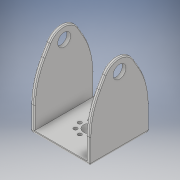
# Autodesk Inventor part: Wheel Case
Saved by Autodesk Inventor 2019 (Build 230136000, 136)
## iProperties
Created: 2018-12-01
Part Number: Wheel Case
Material: Generic
Document SubType Name: Modeling
Designer: Ashley
Density: 1 g/cm^3
Appearance: Default
Author: Ashley
Autodesk Inventor part; units mm, degrees
ref_plane "YZ Plane" through (0, 0, 0) normal (1, 0, 0) x (0, 1, 0)
ref_plane "XZ Plane" through (0, 0, 0) normal (0, 1, 0) x (-1, 0, 0)
ref_plane "XY Plane" through (0, 0, 0) normal (0, 0, 1) x (1, 0, 0)
sketch "Sketch1" plane through (0, 0, 0) normal (0, 1, 0) x (-1, 0, 0)
  line L0 (32.5, 32.5) -> (-32.5, 32.5)
  line L1 (-32.5, 32.5) -> (-32.5, -32.5)
  line L2 (-32.5, -32.5) -> (32.5, -32.5)
  line L3 (32.5, -32.5) -> (32.5, 32.5)
  line L4 (32.5, 32.5) -> (-32.5, -32.5) construction
  line L5 (-32.5, 32.5) -> (32.5, -32.5) construction
  point P0 (0, 0)
  dimension "d0" = 65
  dimension "d1" = 65
  constraints: 12 end point, 2 midpoint, 2 parallel, 1 horizontal, 1 perpendicular
  measures "d0" distance of L1.end L2.end
  measures "d1" distance of L0.end L1.end
extrude "Top Base Extrusion" add sketch "Sketch1" along normal blind 4
sketch "Sketch2" plane through (0, 4, 0) normal (0, 1, 0) x (1, 0, 0)
  line L0 (-32.5, -32.5) -> (32.5, -32.5) construction
  line L1 (32.5, -32.5) -> (32.5, 32.5) construction
  line L2 (-32.5, 32.5) -> (-32.5, -32.5) construction
  line L3 (-32.5, 32.5) -> (-28.5, 32.5)
  line L4 (-28.5, 32.5) -> (-28.5, -32.5)
  line L5 (-28.5, -32.5) -> (-32.5, -32.5)
  line L6 (-32.5, -32.5) -> (-32.5, 32.5)
  line L7 (32.5, 32.5) -> (28.5, 32.5)
  line L8 (28.5, 32.5) -> (28.5, -32.5)
  line L9 (28.5, -32.5) -> (32.5, -32.5)
  line L10 (32.5, -32.5) -> (32.5, 32.5)
  point P0 (0, 0)
  dimension "d4" = 4
  dimension "d5" = 4
  constraints: 16 end point, 4 parallel, 2 horizontal, 2 perpendicular, 2 point on line
  measures "d4" distance between parallel lines of L4 L2
  measures "d5" distance between parallel lines of L1 L8
extrude "Side Extrusions" add sketch "Sketch2" along normal blind 83.6
sketch "Sketch3" plane through (32.5, 0, 32.5) normal (1, 0, 0) x (0, 0, -1)
  circle A0 centre (32.5, 74.5) radius 7.1
  point P0 (32.5, 0)
  dimension "d8" = 14.2
  dimension "d11" = 74.5
  constraints: 1 centre point
  measures "d8" diameter of A0
  measures "d11" distance of point (32.5, 0) A0.centre
extrude "Wheel Axel Hole" cut sketch "Sketch3" against normal up to surface (65 mm away)
sketch "Sketch4" plane through (0, 0, 0) normal (0, -1, 0) x (1, 0, 0)
  circle A0 centre (0, 0) radius 7.1
  circle A1 centre (0, 0) radius 16
  dimension "d16" = 14.2
  dimension "d17" = 32
  constraints: 2 centre point, 2 coincident
  measures "d16" diameter of A0
  measures "d17" diameter of A1
extrude "Chain Interferance Extrusion" add sketch "Sketch4" along normal blind 6
sketch "Sketch5" plane through (0, 0, 0) normal (0, -1, 0) x (1, 0, 0)
  circle A0 centre (0, 0) radius 7.1 construction
  circle A1 centre (0, 0) radius 7.1
  constraints: 1 centre point, 1 coincident, 1 concentric
extrude "Top Center Bearing Hole" cut sketch "Sketch5" against normal up to surface (4 mm away)
sketch "Sketch7" plane through (0, -6, 0) normal (0, -1, 0) x (1, 0, 0)
  circle A0 centre (0, 0) radius 7.1 construction
  circle A1 centre (0, 11.314) radius 2.05
  circle A2 centre (-8.0002, 8.0002) radius 2.05
  circle A3 centre (-11.314, 0) radius 2.05
  circle A4 centre (-8.0002, -8.0002) radius 2.05
  circle A5 centre (0, -11.314) radius 2.05
  circle A6 centre (8.0002, -8.0002) radius 2.05
  circle A7 centre (11.314, 0) radius 2.05
  circle A8 centre (8.0002, 8.0002) radius 2.05
  dimension "d23" = 4.1
  dimension "d24" = 11.314
  dimension "d27" = 360
  constraints: 8 centre point, 17 other
  measures "d23" diameter of A1
  measures "d24" distance of A0.centre A1.centre
extrude "Sprocket Screws Holes" cut sketch "Sketch7" against normal up to next
sketch "Sketch8" plane through (32.5, 0, 32.5) normal (1, 0, 0) x (0, 0, -1)
  line L0 (65, 0) -> (65, 87.6) construction
  line L1 (0, 87.6) -> (65, 87.6) construction
  line L2 (0, 0) -> (0, 87.6) construction
  line L3 (65, 49.2769) -> (42.8742, 87.6)
  line L4 (65, 87.6) -> (0, 87.6) construction
  line L5 (65, 49.2769) -> (109.2517, 49.2769) construction
  line L6 (0, 49.2769) -> (45.0213, 49.2769) construction
  line L7 (0, 49.2769) -> (44.4453, 49.2769) construction
  line L8 (0, 49.2769) -> (22.1258, 87.6)
  line L9 (65, 49.2769) -> (65, 87.6)
  line L10 (42.8742, 87.6) -> (65, 87.6)
  line L11 (22.1258, 87.6) -> (0, 87.6)
  line L12 (0, 49.2769) -> (0, 87.6)
  point P0 (32.5, 0)
  dimension "d32" = 120
  constraints: 18 end point, 4 point on line, 3 collinear, 3 horizontal, 1 equal length, 1 perpendicular
  measures "d32" angle of L5 L3
extrude "Extrusion7" cut sketch "Sketch8" against normal up to surface (65 mm away)
fillet "Fillet1" radius 80 4 edges at (30.5, 49.2769, 32.5) (-30.5, 49.2769, 32.5) (30.5, 49.2769, -32.5) (-30.5, 49.2769, -32.5)
fillet "Fillet2" radius 18 4 edges at (30.5, 87.6, 10.3742) (30.5, 87.6, -10.3742) (-30.5, 87.6, -10.3742) (-30.5, 87.6, 10.3742)
fillet "Fillet3" radius 3 4 edges at (0, 0, -32.5) (-32.5, 0, 0) (32.5, 0, 0) (0, 0, 32.5)
fillet "Fillet4" radius 3 1 edges at (-16, 0, 0)
fillet "Fillet5" radius 1 1 edges at (-16, -6, 0)
fillet "Fillet6" radius 1 32 edges at (32.5, 48.5465, -29.7741) (32.5, 73.2055, -18.6848) (32.5, 87.5696, 0) (32.5, 73.2055, 18.6848) (32.5, 48.5465, 29.7741) (32.5, 15.4205, 32.5) (31.6213, 0.8787, 31.6213) (31.6213, 0.8787, -31.6213) (32.5, 15.4205, -32.5) (28.5, 48.5465, -29.7741) (28.5, 73.2055, -18.6848) (28.5, 87.5696, 0) (28.5, 73.2055, 18.6848) (28.5, 48.5465, 29.7741) (28.5, 15.9205, 32.5) (28.5, 15.9205, -32.5) (-28.5, 48.5465, -29.7741) (-28.5, 73.2055, -18.6848) (-28.5, 87.5696, 0) (-28.5, 73.2055, 18.6848) (-28.5, 48.5465, 29.7741) (-28.5, 15.9205, 32.5) (-28.5, 15.9205, -32.5) (-32.5, 48.5465, -29.7741) (-32.5, 73.2055, -18.6848) (-32.5, 87.5696, 0) (-32.5, 73.2055, 18.6848) (-32.5, 48.5465, 29.7741) (-32.5, 15.4205, 32.5) (-31.6213, 0.8787, 31.6213) (-31.6213, 0.8787, -31.6213) (-32.5, 15.4205, -32.5)
body "Solid1"
